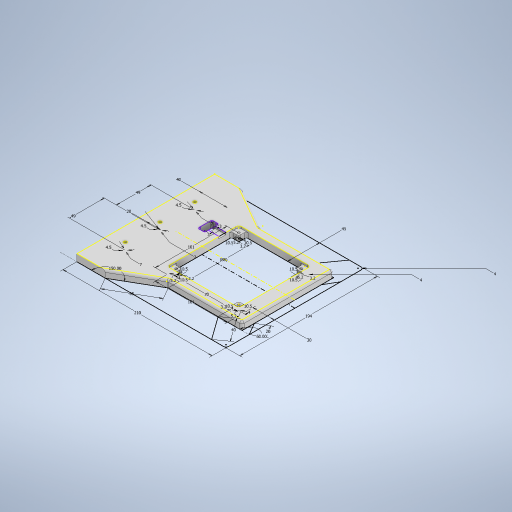
# Autodesk Inventor part: XY_STAGE_BOARD1
Saved by Autodesk Inventor 2023 (Build 270158000, 158)
## iProperties
Created: 2023-08-21
Part Number: XY_STAGE_BOARD1
Material: 일반
Document SubType Name: Modeling
Designer: rlatk
Density: 1 g/cm^3
Appearance: 기본값
Author: rlatk
Autodesk Inventor part; units mm, degrees
ref_plane "YZ Plane" through (0, 0, 0) normal (1, 0, 0) x (0, 1, 0)
ref_plane "XZ Plane" through (0, 0, 0) normal (0, 1, 0) x (-1, 0, 0)
ref_plane "XY Plane" through (0, 0, 0) normal (0, 0, 1) x (1, 0, 0)
sketch "스케치1" plane through (0, 0, 0) normal (0, 1, 0) x (-1, 0, 0)
  line L0 (0, 0) -> (-206, 0)
  line L1 (-210, 4) -> (-210, 190)
  line L2 (-206, 194) -> (0, 194)
  line L3 (0, 194) -> (0, 0)
  line L4 (-40, 0) -> (-40, 194)
  line L5 (-20, 0) -> (-20, 194)
  circle A0 centre (-20, 97) radius 3.5
  circle A1 centre (-20, 48) radius 3.5
  circle A2 centre (-20, 146) radius 3.5
  arc A3 (-210, 4) -> (-206, 0) centre (-206, 4) ccw
  arc A4 (-206, 194) -> (-210, 190) centre (-206, 190) ccw
  circle A5 centre (-20, 97) radius 2.25
  circle A6 centre (-20, 146) radius 2.25
  circle A7 centre (-20, 48) radius 2.25
  line L6 (-40, 194) -> (-96.2917, 161.5)
  line L7 (-40, 194) -> (25, 194) construction
  line L8 (-96.2917, 161.5) -> (-166.2917, 161.5)
  line L9 (-166.2917, 161.5) -> (-189.6101, 194)
  line L10 (-210, 161.5) -> (-200, 144.1795)
  line L11 (-210, 161.5) -> (-190, 161.5) construction
  line L12 (-210, 97) -> (-40, 97)
  line L13 (-40, 0) -> (-96.2917, 32.5)
  line L14 (-96.2917, 32.5) -> (-166.2917, 32.5)
  line L15 (-166.2917, 32.5) -> (-189.6101, 0)
  line L16 (-210, 32.5) -> (-200, 49.8205)
  line L17 (-200, 144.1795) -> (-200, 49.8205)
  line L18 (-166.2917, 32.5) -> (-200, 32.5)
  line L19 (-200, 32.5) -> (-200, 49.8205)
  line L20 (-200, 144.1795) -> (-200, 161.5)
  line L21 (-166.2917, 161.5) -> (-200, 161.5)
  point P0 (-210, 194)
  point P1 (-210, 0)
  dimension "d0" = 210
  dimension "d1" = 194
  dimension "d2" = 40
  dimension "d3" = 20
  dimension "d4" = 7
  dimension "d5" = 7
  dimension "d6" = 7
  dimension "d7" = 49
  dimension "d8" = 49
  dimension "d9" = 4
  dimension "d17" = 4.5
  dimension "d18" = 4.5
  dimension "d19" = 4.5
  dimension "d82" = 65
  dimension "d83" = 150
  dimension "d84" = 70
  dimension "d85" = 40
  dimension "d86" = 20
  dimension "d87" = 60
  constraints: 44 end point, 12 point on line, 8 centre point, 5 horizontal, 5 symmetric about line, 4 midpoint, 4 perpendicular, 4 point on circle, 4 tangent, 3 coincident, 2 equal length, 2 parallel, 1 collinear, 1 equal radius, 1 vertical
  measures "d0" distance of point (-210, 194) L2.end
  measures "d1" distance of point (-210, 0) point (-210, 194)
  measures "d2" distance between parallel lines of L3 L4
  measures "d3" distance between parallel lines of L3 L5
  measures "d4" diameter of A0
  measures "d5" diameter of A1
  measures "d6" diameter of A2
  measures "d7" distance of A1.centre A0.centre
  measures "d8" distance of A2.centre A0.centre
  measures "d9" radius of A3
  measures "d17" diameter of A5
  measures "d18" diameter of A6
  measures "d19" diameter of A7
  measures "d82" distance of L4.end L6.end
  measures "d83" angle of L6 L7
  measures "d84" distance of L6.end L8.end
  measures "d85" distance of L8.end L9.end
  measures "d86" distance of L10.start L10.end
  measures "d87" angle of L10 L11
extrude "돌출1" add sketch "스케치1" along normal blind 10
extrude "돌출2" cut sketch "스케치1" along normal blind 3 contours A1 L5 A7 | L5 A7 A1 | A7 L5 | L5 A7 | A2 L5 A6 | L5 A6 A2 | A0 L5 A5 | L5 A5 A0 | A6 L5 | L5 A6 | A5 L5 | L5 A5
sketch "스케치2" plane through (0, 0, 0) normal (0, -1, 0) x (1, 0, 0)
  line L0 (176, 45) -> (83, 45)
  line L1 (79, 49) -> (79, 142)
  line L2 (83, 146) -> (176, 146)
  line L3 (180, 142) -> (180, 49)
  line L4 (206, 0) -> (0, 0) projected
  line L5 (210, 190) -> (210, 4) projected
  arc A0 (176, 45) -> (180, 49) centre (176, 49) ccw
  arc A1 (180, 142) -> (176, 146) centre (176, 142) ccw
  arc A2 (83, 146) -> (79, 142) centre (83, 142) ccw
  arc A3 (79, 49) -> (83, 45) centre (83, 49) ccw
  line L6 (180, 45) -> (169.5, 45)
  line L7 (169.5, 45) -> (169.5, 55.5)
  line L8 (169.5, 55.5) -> (180, 55.5)
  line L9 (180, 55.5) -> (180, 45)
  line L10 (79, 45) -> (89.5, 45)
  line L11 (89.5, 45) -> (89.5, 55.5)
  line L12 (89.5, 55.5) -> (79, 55.5)
  line L13 (79, 55.5) -> (79, 45)
  line L14 (180, 146) -> (169.5, 146)
  line L15 (169.5, 146) -> (169.5, 135.5)
  line L16 (169.5, 135.5) -> (180, 135.5)
  line L17 (180, 135.5) -> (180, 146)
  line L18 (79, 146) -> (89.5, 146)
  line L19 (89.5, 146) -> (89.5, 135.5)
  line L20 (89.5, 135.5) -> (79, 135.5)
  line L21 (79, 135.5) -> (79, 146)
  circle A4 centre (173.5, 51.5) radius 1.6
  circle A5 centre (85.5, 51.5) radius 1.6
  circle A6 centre (85.5, 139.5) radius 1.6
  circle A7 centre (173.5, 139.5) radius 1.6
  line L22 (173.5, 51.5) -> (169.5, 51.5)
  line L23 (170.4978, 51.5) -> (171.9989, 54.1)
  line L24 (171.9989, 54.1) -> (175.0011, 54.1)
  line L25 (175.0011, 54.1) -> (176.5022, 51.5)
  line L26 (176.5022, 51.5) -> (175.0011, 48.9)
  line L27 (175.0011, 48.9) -> (171.9989, 48.9)
  line L28 (171.9989, 48.9) -> (170.4978, 51.5)
  line L29 (85.5, 51.5) -> (89.5, 51.5)
  line L30 (88.5022, 51.5) -> (87.0011, 48.9)
  line L31 (87.0011, 48.9) -> (83.9989, 48.9)
  line L32 (83.9989, 48.9) -> (82.4978, 51.5)
  line L33 (82.4978, 51.5) -> (83.9989, 54.1)
  line L34 (83.9989, 54.1) -> (87.0011, 54.1)
  line L35 (87.0011, 54.1) -> (88.5022, 51.5)
  line L36 (85.5, 139.5) -> (89.5, 139.5)
  line L37 (88.5022, 139.5) -> (87.0011, 136.9)
  line L38 (87.0011, 136.9) -> (83.9989, 136.9)
  line L39 (83.9989, 136.9) -> (82.4978, 139.5)
  line L40 (82.4978, 139.5) -> (83.9989, 142.1)
  line L41 (83.9989, 142.1) -> (87.0011, 142.1)
  line L42 (87.0011, 142.1) -> (88.5022, 139.5)
  line L43 (173.5, 139.5) -> (169.5, 139.5)
  line L44 (170.4978, 139.5) -> (171.9989, 142.1)
  line L45 (171.9989, 142.1) -> (175.0011, 142.1)
  line L46 (175.0011, 142.1) -> (176.5022, 139.5)
  line L47 (176.5022, 139.5) -> (175.0011, 136.9)
  line L48 (175.0011, 136.9) -> (171.9989, 136.9)
  line L49 (171.9989, 136.9) -> (170.4978, 139.5)
  point P0 (174.75, 55.5)
  dimension "d14" = 101
  dimension "d15" = 101
  dimension "d16" = 45
  dimension "d24" = 30
  dimension "d25" = 4
  dimension "d26" = 10.5
  dimension "d27" = 10.5
  dimension "d28" = 10.5
  dimension "d29" = 10.5
  dimension "d30" = 10.5
  dimension "d31" = 10.5
  dimension "d32" = 10.5
  dimension "d33" = 10.5
  dimension "d34" = 3.2
  dimension "d36" = 4
  dimension "d37" = 3.2
  dimension "d38" = 4
  dimension "d39" = 4
  dimension "d40" = 3.2
  dimension "d41" = 4
  dimension "d42" = 4
  dimension "d43" = 3.2
  dimension "d44" = 4
  dimension "d45" = 4
  dimension "d46" = 4
  dimension "d58" = 5.2
  dimension "d59" = 5.2
  dimension "d60" = 5.2
  dimension "d61" = 5.2
  dimension "d95" = 88
  constraints: 96 end point, 16 point on line, 10 parallel, 9 perpendicular, 8 centre point, 8 point on circle, 8 tangent, 5 horizontal, 4 coincident, 3 equal radius, 1 midpoint, 52 other
  measures "d14" distance of L18.start L14.start
  measures "d15" distance of L10.start L18.start
  measures "d16" distance between parallel lines of L4 L0
  measures "d24" distance between parallel lines of L5 L3
  measures "d25" radius of A0
  measures "d26" distance of L7.end L8.end
  measures "d27" distance of L6.end L7.end
  measures "d28" distance of L12.end L11.end
  measures "d29" distance of L11.end L10.end
  measures "d30" distance of L16.end L15.end
  measures "d31" distance of L15.end L14.end
  measures "d32" distance of L19.end L20.end
  measures "d33" distance of L18.end L19.end
  measures "d34" diameter of A4
  measures "d36" distance from line of L7 L22.start
  measures "d37" diameter of A5
  measures "d38" distance from line of L11 L29.start
  measures "d39" distance from line of L12 L29.start
  measures "d40" diameter of A6
  measures "d41" distance from line of L20 L36.start
  measures "d42" distance from line of L19 L36.start
  measures "d43" diameter of A7
  measures "d44" distance from line of L15 L43.start
  measures "d45" distance from line of L16 L43.start
  measures "d46" distance from line of L8 L22.start
  measures "d58" distance between parallel lines of L23 L26
  measures "d59" distance between parallel lines of L33 L30
  measures "d60" distance between parallel lines of L40 L37
  measures "d61" distance between parallel lines of L44 L47
  measures "d95" distance of L29.start L36.start
extrude "돌출3" cut sketch "스케치1" along normal blind 4 contours A1 L5 A7 | L5 A7 A1 | A7 L5 | L5 A7 | A2 L5 A6 | L5 A6 A2 | A0 L5 A5 | L5 A5 A0 | A6 L5 | L5 A6 | A5 L5 | L5 A5
extrude "돌출4" cut sketch "스케치1" along normal blind 10 contours A7 L5 | L5 A7 | A6 L5 | L5 A6 | A5 L5 | L5 A5
sketch "스케치4" plane through (0, 10, 0) normal (0, 1, 0) x (1, 0, 0)
  line L0 (176, -45) -> (83, -45) projected
  line L1 (180, -142) -> (180, -49) projected
  line L2 (79, -49) -> (79, -142) projected
  line L3 (83, -146) -> (176, -146) projected
  line L4 (79, -135.5) -> (79, -146) projected
  line L5 (79, -146) -> (89.5, -146) projected
  line L6 (180, -135.5) -> (180, -146) projected
  line L7 (180, -146) -> (169.5, -146) projected
  line L8 (180, -45) -> (169.5, -45) projected
  line L9 (180, -55.5) -> (180, -45) projected
  line L10 (79, -45) -> (89.5, -45) projected
  line L11 (79, -55.5) -> (79, -45) projected
  arc A0 (83, -45) -> (79, -49) centre (83, -49) ccw projected
  arc A1 (180, -49) -> (176, -45) centre (176, -49) ccw projected
  arc A2 (176, -146) -> (180, -142) centre (176, -142) ccw projected
  arc A3 (79, -142) -> (83, -146) centre (83, -142) ccw projected
  point P0 (0, 0)
extrude "돌출6" cut sketch "스케치4" against normal blind 3 contours A1 L1 A2 L3 A3 L2 A0 L0
extrude "돌출7" cut sketch "스케치2" against normal blind 10 contours A4 | A5 | A7 | A6
extrude "돌출8" cut sketch "스케치2" against normal blind 2 contours A4 | L23 L24 L25 L26 L27 L28 | A5 | L30 L31 L32 L33 L34 L35 | A7 | L44 L45 L46 L47 L48 L49 | A6 | L37 L38 L39 L40 L41 L42
sketch "스케치5" plane through (0, 7, 0) normal (0, 1, 0) x (1, 0, 0)
  line L0 (89.5, -55.5) -> (79, -55.5) projected
  line L1 (89.5, -45) -> (89.5, -55.5) projected
  line L2 (176, -45) -> (83, -45) projected
  line L3 (169.5, -45) -> (169.5, -55.5) projected
  line L4 (169.5, -55.5) -> (180, -55.5) projected
  line L5 (180, -142) -> (180, -49) projected
  line L6 (169.5, -135.5) -> (180, -135.5) projected
  line L7 (169.5, -146) -> (169.5, -135.5) projected
  line L8 (83, -146) -> (176, -146) projected
  line L9 (89.5, -146) -> (89.5, -135.5) projected
  line L10 (89.5, -135.5) -> (79, -135.5) projected
  line L11 (79, -49) -> (79, -142) projected
  point P0 (0, 0)
extrude "돌출9" cut sketch "스케치5" against normal blind 10
fillet "모깎기2" radius 3 12 edges at (169.5, 3.5, 55.5) (169.5, 3.5, 45) (180, 3.5, 55.5) (180, 3.5, 135.5) (169.5, 3.5, 135.5) (169.5, 3.5, 146) (89.5, 3.5, 146) (89.5, 3.5, 135.5) (79, 3.5, 135.5) (89.5, 3.5, 45) (79, 3.5, 55.5) (89.5, 3.5, 55.5)
extrude "돌출14" cut sketch "스케치1" along normal blind 10 contours L0 L15 L14 L13 | L6 L8 L9 L2
extrude "돌출15" cut sketch "스케치1" along normal blind 10 contours L17 L16 L1 L12 | L12 L1 L10 L17
extrude "돌출16" cut sketch "스케치1" along normal blind 10 contours L0 A3 L1 L16 L19 L18 L15 | L9 L21 L20 L10 L1 A4 L2
fillet "모깎기5" radius 3 9 edges at (200, 5, 32.5) (200, 5, 161.5) (148.1458, 10, 32.5) (200, 10, 97) (148.1458, 10, 161.5) (68.1458, 10, 16.25) (96.2917, 5, 32.5) (96.2917, 5, 161.5) (68.1458, 10, 177.75)
sketch "스케치11" plane through (0, 10, 0) normal (0, 1, 0) x (1, 0, 0)
  line L0 (34, 0) -> (94.0955, -34.6962) projected
  line L1 (34, 0) -> (0, 0) projected
  line L2 (0, 0) -> (0, -194) projected
  line L3 (0, -194) -> (34, -194) projected
  line L4 (94.0955, -159.3038) -> (34, -194) projected
  arc A0 (97.0955, -158.5) -> (94.0955, -159.3038) centre (97.0955, -164.5) ccw projected
  line L5 (197, -158.5) -> (97.0955, -158.5) projected
  line L6 (197, -35.5) -> (197, -158.5) projected
  line L7 (97.0955, -35.5) -> (197, -35.5) projected
  arc A1 (94.0955, -34.6962) -> (97.0955, -35.5) centre (97.0955, -29.5) ccw projected
  circle A2 centre (20, -48) radius 2.25 projected
  circle A3 centre (20, -97) radius 2.25 projected
  circle A4 centre (20, -146) radius 2.25 projected
  arc A5 (176, -146) -> (180, -142) centre (176, -142) ccw projected
  line L8 (176, -146) -> (83, -146) projected
  arc A6 (79, -142) -> (83, -146) centre (83, -142) ccw projected
  line L9 (79, -142) -> (79, -49) projected
  arc A7 (83, -45) -> (79, -49) centre (83, -49) ccw projected
  line L10 (83, -45) -> (176, -45) projected
  arc A8 (180, -49) -> (176, -45) centre (176, -49) ccw projected
  line L11 (180, -49) -> (180, -142) projected
  line L12 (210, -97) -> (40, -97) projected
  arc A9 (54, -76) -> (56, -78) centre (56, -76) ccw
  line L13 (56, -78) -> (62, -78)
  arc A10 (62, -78) -> (64, -76) centre (62, -76) ccw
  line L14 (64, -76) -> (64, -60)
  arc A11 (64, -60) -> (62, -58) centre (62, -60) ccw
  line L15 (62, -58) -> (56, -58)
  arc A12 (56, -58) -> (54, -60) centre (56, -60) ccw
  line L16 (54, -60) -> (54, -76)
  line L17 (79, -58.5) -> (79, -132.5) projected
  line L18 (79, -73) -> (64, -73)
  line L19 (64, -73) -> (64, -63)
  line L20 (64, -63) -> (79, -63)
  line L21 (79, -63) -> (79, -73)
  dimension "d104" = 3
  dimension "d105" = 3
  constraints: 16 end point, 8 point on circle, 4 centre point, 2 parallel, 2 point on line, 1 horizontal, 1 perpendicular
  measures "d104" distance from line of L14.start L18
  measures "d105" distance of L14.end L19.end
extrude "돌출19" cut sketch "스케치11" against normal blind 3 contours L18 L14 L20 L9
extrude "돌출20" cut sketch "스케치11" against normal blind 10 contours L14 A10 L13 A9 L16 A12 L15 A11
